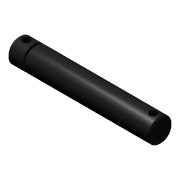
# Autodesk Inventor part: pino_a3
Saved by Autodesk Inventor 2012 SP2 (Build 160219200, 219)
## iProperties
Created: 2015-05-25
Part Number: pino_a3
Material: Aço carbono
Document SubType Name: Modeling
Designer: Projeto02
Density: 7.87 g/cm^3
Mass: 31.1389 g
Surface Area: 19.5859 cm^2
Volume: 3.95665 cm^3
Author: Projeto02
Autodesk Inventor part; units mm, degrees
ref_plane "YZ Plane" through (0, 0, 0) normal (1, 0, 0) x (0, 1, 0)
ref_plane "XZ Plane" through (0, 0, 0) normal (0, 1, 0) x (-1, 0, 0)
ref_plane "XY Plane" through (0, 0, 0) normal (0, 0, 1) x (1, 0, 0)
sketch "Esboço2" plane through (0, 0, 0) normal (1, 0, 0) x (0, 1, 0)
  circle A0 centre (0, 0) radius 4.7625
  dimension "d0" = 9.525
  constraints: 1 centre point, 1 coincident
  measures "d0" diameter of A0
extrude "Extrusão1" add sketch "Esboço2" along normal blind 6
sketch "Esboço3" plane through (6, 0, 0) normal (1, 0, 0) x (0, 0, -1)
  circle A0 centre (0, 0) radius 4.7625 projected
  circle A1 centre (0, 0) radius 3.5719
  dimension "d3" = 7.1437
  constraints: 1 centre point, 1 coincident
  measures "d3" diameter of A1
extrude "Extrusão2" add sketch "Esboço3" along normal blind 1 contours A1
sketch "Esboço4" plane through (7, 0, 0) normal (1, 0, 0) x (0, 0, -1)
  circle A0 centre (0, 0) radius 3.5719 projected
  circle A1 centre (0, 0) radius 4.7625
  dimension "d6" = 9.525
  constraints: 1 centre point, 1 coincident
  measures "d6" diameter of A1
extrude "Extrusão3" add sketch "Esboço4" along normal blind 50 contours A0 | A1
chamfer "Chanfro1" distance 0.5 angle 45 2 edges at (0, -4.7625, 0) (57, 0, 4.7625)
sketch "Esboço7" plane through (0, 0, 0) normal (0, 0, 1) x (1, 0, 0)
  line L0 (57, 4.2625) -> (57, -4.2625) projected
  line L1 (0, -4.2625) -> (0, 4.2625) projected
  point P0 (0, 0)
  point P1 (54, 0)
  point P2 (3, 0)
  dimension "d18" = 3
  dimension "d33" = 3
  constraints: 1 horizontal alignment
  measures "d18" distance from line of L0 point (54, 0)
  measures "d33" distance from line of point (3, 0) L1
hole "Furo1" at (54, 0, 0) at (3, 0, 0) direction (0, 0, -1) diameter 3 end through all
hole "Furo2" at (54, 0, 0) at (3, 0, 0) direction (0, 0, 1) diameter 3 end through all
equation "\"d33\" = d18"
